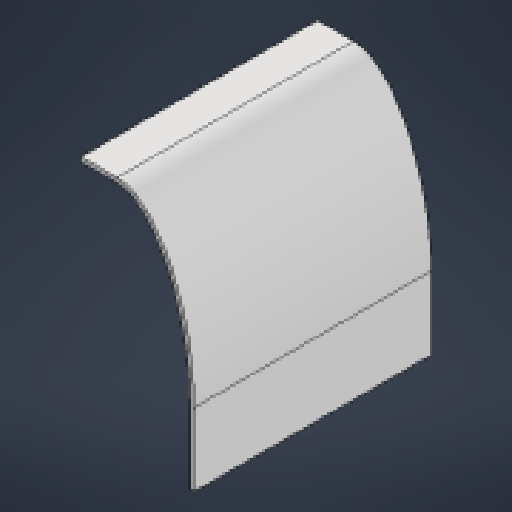
# Autodesk Inventor part: Intake hood polycarb
Saved by Autodesk Inventor 2023.2 (Build 272271030, 271C)
## iProperties
Created: 2023-04-04
Part Number: Intake hood polycarb
Material: Generic
Document SubType Name: Modeling
Designer: Main Account
Density: 1 g/cm^3
Appearance: Default
Author: Main Account
Autodesk Inventor part; units mm, degrees
ref_plane "YZ Plane" through (0, 0, 0) normal (1, 0, 0) x (0, 1, 0)
ref_plane "XZ Plane" through (0, 0, 0) normal (0, 1, 0) x (-1, 0, 0)
ref_plane "XY Plane" through (0, 0, 0) normal (0, 0, 1) x (1, 0, 0)
sketch "Sketch1" plane through (0, 0, 0) normal (0, 0, 1) x (1, 0, 0)
  line L0 (-52.1863, 17.4625) -> (-39.6331, 17.4625)
  ellipse E0 centre (-35.0357, -29.0502) end of major axis (-40.9054, 17.3827) minor radius 21.7222 (-12.7, -38.6239) -> (-39.6331, 17.4625) ccw
  line L1 (-12.7, -38.6239) -> (-12.7, -64.0239)
  line L2 (-52.1863, 15.875) -> (-39.6331, 15.875)
  line L3 (-14.2875, -38.6239) -> (-14.2875, -64.0239)
  line L4 (-52.1863, 17.4625) -> (-52.1863, 15.875)
  line L5 (-12.7, -64.0239) -> (-14.2875, -64.0239)
  spline S0 degree 5 poles (-39.6331, 15.8751) (-39.5506, 15.8751) (-39.4681, 15.8741) (-39.3857, 15.8721) (-38.0942, 15.8262) (-36.8136, 15.5443) (-35.6732, 15.1037) (-33.1533, 13.7975) (-30.9609, 11.9793) (-29.8061, 10.841) (-27.3673, 8.0794) (-25.3083, 5.0217) (-24.2528, 3.2489) (-22.1488, -0.7015) (-20.41, -4.8272) (-19.5649, -7.0886) (-17.9813, -11.8632) (-16.7471, -16.7402) (-16.1934, -19.2984) (-15.2526, -24.4756) (-14.6572, -29.7039) (-14.4448, -32.341) (-14.3123, -35.1828) (-14.2891, -38.0258) (-14.288, -38.2252) (-14.2875, -38.4245) (-14.2875, -38.6239) knots 0 0 0 0 0 0 0.006424 0.006424 0.006424 0.10063 0.10063 0.10063 0.226594 0.226594 0.226594 0.387029 0.387029 0.387029 0.574874 0.574874 0.574874 0.778571 0.778571 0.778571 0.984473 0.984473 0.984473 1 1 1 1 1 1
  point P0 (0, 0)
  dimension "d2" = 1.5875
  dimension "d1" = 25.4
  constraints: 12 end point, 3 horizontal, 2 parallel, 2 vertical, 1 perpendicular, 7 other
  measures "d1" distance of L1.start L1.end
extrude "Extrusion1" add sketch "Sketch1" against normal blind 82.55
body "Solid1"
